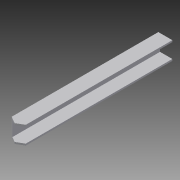
# Autodesk Inventor part: Chassis Cross Support
Saved by Autodesk Inventor 2013 (Build 170138000, 138)
## iProperties
Created: 2013-01-29
Part Number: Chassis Cross Support
Material: Generic
Document SubType Name: Modeling
Designer: carneeki
Density: 1 g/cm^3
Author: carneeki
Autodesk Inventor part; units mm, degrees
ref_plane "YZ Plane" through (0, 0, 0) normal (1, 0, 0) x (0, 1, 0)
ref_plane "XZ Plane" through (0, 0, 0) normal (0, 1, 0) x (-1, 0, 0)
ref_plane "XY Plane" through (0, 0, 0) normal (0, 0, 1) x (1, 0, 0)
sketch "Sketch2" plane through (0, 0, 0) normal (0, 0, 1) x (1, 0, 0)
  line L0 (0, 0) -> (0, 32)
  line L1 (0, 32) -> (25, 32)
  line L2 (25, 32) -> (25, 29)
  line L3 (25, 29) -> (3, 29)
  line L4 (3, 29) -> (3, 3)
  line L5 (3, 3) -> (25, 3)
  line L6 (25, 3) -> (25, 0)
  line L7 (25, 0) -> (0, 0)
  dimension "d10" = 22
  dimension "d11" = 25
  dimension "d12" = 26
  dimension "d13" = 3
  dimension "d14" = 29
  dimension "d15" = 25
  dimension "d16" = 29
  dimension "d17" = 0
  constraints: 16 end point, 6 parallel, 1 horizontal, 1 perpendicular
  measures "d10" distance between parallel lines of L2 L4
  measures "d11" distance between parallel lines of L0 L2
  measures "d12" distance between parallel lines of L3 L5
  measures "d13" distance between parallel lines of L1 L3
  measures "d14" distance between parallel lines of L3 L7
  measures "d15" distance from line of point (0, 0) L2
  measures "d16" distance from line of point (0, 0) L3
  measures "d17" distance between parallel lines of L6 L2
extrude "Extrusion1" add sketch "Sketch2" against normal blind 268.3002
chamfer "Chamfer1" distance 12.5 angle 30 1 edges at (0, 16, 0) measured on face at (0.5, 16, 0)
chamfer "Chamfer2" distance 12.5 angle 30 1 edges at (25, 30.5, 0) measured on face at (24.5, 30.5, 0)
chamfer "Chamfer6" distance 12.5 angle 30 1 edges at (25, 1.5, 0) measured on face at (24.5, 1.5, 0)
body "Solid1"
